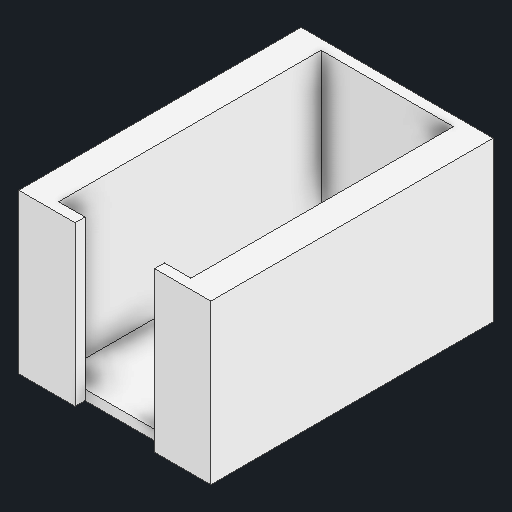
# Autodesk Inventor part: HorizontalRotationServoHolder
Saved by Autodesk Inventor 2025 (Build 290162000, 162)
## iProperties
Created: 2024-04-23
Part Number: HorizontalRotationServoHolder
Material: Generic
Document SubType Name: Modeling
Designer: conno
Density: 1 g/cm^3
Appearance: Default
Author: conno
Autodesk Inventor part; units mm, degrees
ref_plane "YZ Plane" through (0, 0, 0) normal (1, 0, 0) x (0, 1, 0)
ref_plane "XZ Plane" through (0, 0, 0) normal (0, 1, 0) x (-1, 0, 0)
ref_plane "XY Plane" through (0, 0, 0) normal (0, 0, 1) x (1, 0, 0)
sketch "Sketch1" plane through (0, 0, 0) normal (0, 1, 0) x (-1, 0, 0)
  line L0 (9.779, 20.1676) -> (-9.779, 20.1676)
  line L1 (-9.779, 20.1676) -> (-9.779, -20.1676)
  line L2 (-9.779, -20.1676) -> (9.779, -20.1676)
  line L3 (9.779, -20.1676) -> (9.779, 20.1676)
  line L4 (9.779, 20.1676) -> (-9.779, -20.1676) construction
  line L5 (-9.779, 20.1676) -> (9.779, -20.1676) construction
  point P0 (0, 0)
  dimension "d0" = 19.558
  dimension "d1" = 40.3352
  constraints: 12 end point, 2 midpoint, 2 parallel, 1 horizontal, 1 perpendicular
  measures "d0" distance of L2.end L1.end
  measures "d1" distance of L1.end L0.end
extrude "Base" add sketch "Sketch1" along normal blind 1.5875
thicken "Outward Servo Body Offset" operation add thickness 0.7937 both sides no extend neighbours no toward (0, 0, 1) faces at (-3.2597, 0.5292, 20.1676) (9.779, 1.0583, 6.7225) (3.2597, 0.5292, -20.1676) (-9.779, 1.0583, -6.7225)
sketch "Sketch3" plane through (0, 0, 0) normal (0, -1, 0) x (1, 0, 0)
  line L0 (10.5727, -20.9614) -> (-10.5728, -20.9613) projected
  line L1 (-10.5728, -20.9613) -> (-10.5727, 20.9614) projected
  line L2 (-10.5727, 20.9614) -> (10.5727, 20.9614) projected
  line L3 (10.5727, 20.9614) -> (10.5727, -20.9614) projected
  line L4 (-12.1603, -22.5489) -> (12.1603, -22.5489)
  line L5 (12.1603, -22.5489) -> (12.1603, 22.5488)
  line L6 (12.1603, 22.5488) -> (-12.1603, 22.5488)
  line L7 (-12.1603, 22.5488) -> (-12.1603, -22.5489)
  line L8 (-6.35, 22.5489) -> (-6.35, 20.9614)
  line L9 (6.35, 22.5489) -> (6.35, 20.9614)
  line L10 (-10.5727, 20.9614) -> (10.5727, 20.9614) projected
  point P0 (0, 20.9614)
  dimension "d21" = 1.5875
  dimension "d22" = 12.7
  dimension "d23" = 6.35
  constraints: 12 end point, 4 point on line, 2 perpendicular, 1 midpoint, 3 other
  measures "d21" distance between parallel lines of L0 L4
  measures "d22" distance between parallel lines of L9 L8
  measures "d23" distance from line of point (0, 20.961) L8
extrude "Walls" add sketch "Sketch3" against normal blind 25.4 contours L3 L2 L9 L6 L5 L4 L7 L8 L1 L0
thicken "Right Side Wall Thickening" operation add thickness 3.175 both sides no extend neighbours no toward (1, 0, 0) faces at (12.1603, 8.4667, -7.5163)
thicken "Left Side Wall Thickening" operation add thickness 3.175 both sides no extend neighbours no toward (-1, 0, 0) faces at (-12.1603, 8.4667, 7.5163)
equation "\"d0\" = ServoWidth"
equation "\"d1\" = ServoHeight"
equation "\"d23\" = 0.5 * d22"
equation "\"ServoWidth\" = 19.558"
equation "\"ServoHeight\" = 40.3352"
body "Solid1"
